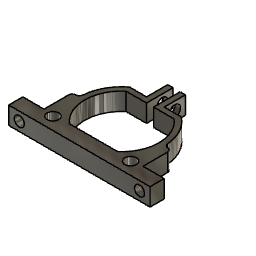
motor unite left v17 (Autodesk Fusion 360 archive; units mm, degrees)
design "motor mount back"
Autodesk Fusion 360 part; units mm, degrees
sketch "スケッチ1" plane through (0, 0, 0) normal (0, 0, 1) x (1, 0, 0)
  line L0 (-14, -12) -> (14, -12)
  line L1 (14, -12) -> (20, -12)
  line L2 (20, -12) -> (20, -8)
  line L3 (20, -8) -> (14, -8)
  line L4 (-14, -12) -> (-20, -12)
  line L5 (-20, -12) -> (-20, -8)
  line L6 (-20, -8) -> (-14, -8)
  line L7 (-14, -8) -> (-14, 0)
  line L8 (14, -8) -> (14, 0)
  circle A0 centre (11, -8.5) radius 1.65
  circle A1 centre (-11, -8.5) radius 1.65
  line L9 (0, 8) -> (-6.8007, 8)
  line L10 (0, 8) -> (6.8007, 8)
  line L11 (0, -8) -> (6.8007, -8)
  line L12 (0, -8) -> (-6.8007, -8)
  arc A2 (-6.8007, 8) -> (-6.8007, -8) centre (0, 0) ccw
  arc A3 (6.8007, -8) -> (6.8007, 8) centre (0, 0) ccw
  line L13 (-14, 0) -> (-12, 0)
  line L14 (12, 0) -> (14, 0)
  line L15 (0, 9.5) -> (7.3314, 9.5)
  line L16 (0, 9.5) -> (-7.3314, 9.5)
  arc A4 (-7.3314, 9.5) -> (-12, 0) centre (0, 0) ccw
  arc A5 (12, 0) -> (7.3314, 9.5) centre (0, 0) ccw
  line L17 (-1, 13.5) -> (-2.5, 13.5)
  line L18 (-2.5, 13.5) -> (-2.5, 9.5)
  line L19 (-1, 13.5) -> (-1, 8)
  line L20 (1, 13.5) -> (1, 8)
  line L21 (1, 13.5) -> (2.5, 13.5)
  line L22 (2.5, 13.5) -> (2.5, 9.5)
  dimension "d223" = 3.3
  constraint perpendicular L1 L2
  constraint perpendicular L4 L5
  constraint perpendicular L6 L7
  constraint perpendicular L3 L8
  constraint coincident A2.centre A3.centre
  constraint perpendicular L7 L13
  constraint perpendicular L8 L14
  constraint parallel L16 L17
  constraint coincident L16 L18.end
  constraint perpendicular L16 L18
  constraint coincident L9 L19.end
  constraint perpendicular L9 L19
  constraint coincident L10 L20.end
  constraint perpendicular L10 L20
  constraint perpendicular L20 L21
  constraint coincident L15 L22.end
  constraint perpendicular L15 L22
  measures "d223" diameter of A0
extrude "押し出し51" add sketch "スケッチ1" along normal blind 5 contours L0 L1 L2 L3 L4 L5 L6 L7 L8 L9 L10 L11 L12 A2 A3 L13 L14 L15 L16 A4 A5 L19 L20 | L16 L17 L18 L19 | L15 L20 L21 L22
extrude "押し出し52" add 2 faces at (-1.5, 13.5, 1.6667) (1.5, 13.5, 1.6667) along direction (0, 1, 0) blind 2
ref_plane "作業平面23" through (2.5, 12.5, 2.5) normal (1, 0, 0) x (0, 1, 0)
sketch "スケッチ26" plane through (2.5, 12.5, 2.5) normal (1, 0, 0) x (0, 1, 0)
  circle A0 centre (0, 0) radius 1.6
  constraint coincident A0.centre origin
extrude "押し出し53" cut sketch "スケッチ26" against normal blind 7
ref_plane "作業平面24" through (17, -8, 2.5) normal (0, 1, 0) x (-1, 0, 0)
sketch "スケッチ27" plane through (17, -8, 2.5) normal (0, 1, 0) x (1, 0, 0)
  circle A0 centre (0, 0) radius 1.6
  dimension "d265" = 3.2
  constraint coincident A0.centre origin
  measures "d265" diameter of A0
extrude "押し出し54" cut sketch "スケッチ27" against normal blind 5
ref_plane "作業平面25" through (-17, -8, 2.5) normal (0, 1, 0) x (-1, 0, 0)
sketch "スケッチ28" plane through (-17, -8, 2.5) normal (0, 1, 0) x (1, 0, 0)
  circle A0 centre (0, 0) radius 1.6
  dimension "d269" = 3.2
  constraint coincident A0.centre origin
  measures "d269" diameter of A0
extrude "押し出し55" cut sketch "スケッチ28" against normal blind 5
fillet "フィレット63" radius 1 1 edges at (-14, 0, 2.5)
fillet "フィレット64" radius 1 1 edges at (-12, 0, 2.5)
fillet "フィレット65" radius 1 1 edges at (12, 0, 2.5)
fillet "フィレット66" radius 1 1 edges at (14, 0, 2.5)
sketch "スケッチ29" plane through (0, -12, 0) normal (0, -1, 0) x (1, 0, 0)
  circle A0 centre (-17, 2.5) radius 1.6
  circle A1 centre (17, 2.5) radius 1.6
  line L0 (-20, 0) -> (20, 0)
  line L1 (20, 0) -> (20, 5)
  line L2 (20, 5) -> (-20, 5)
  line L3 (-20, 5) -> (-20, 0)
  circle A2 centre (-17, 2.5) radius 1.55
  circle A3 centre (17, 2.5) radius 1.55
  dimension "d280" = 3.1
  dimension "d281" = 3.1
  constraint concentric A0 A2
  constraint concentric A1 A3
  measures "d280" diameter of A2
  measures "d281" diameter of A3
extrude "押し出し56" add sketch "スケッチ29" against normal blind 4 contours A0 | A1
sketch "スケッチ30" plane through (0, -12, 0) normal (0, -1, 0) x (1, 0, 0)
  circle A0 centre (17, 2.5) radius 1.55
  circle A1 centre (-17, 2.5) radius 1.55
  line L0 (-20, 0) -> (20, 0)
  line L1 (20, 0) -> (20, 5)
  line L2 (20, 5) -> (-20, 5)
  line L3 (-20, 5) -> (-20, 0)
  circle A2 centre (-17, 2.5) radius 1.425
  circle A3 centre (17, 2.5) radius 1.425
  dimension "d284" = 2.85
  dimension "d285" = 2.85
  constraint concentric A1 A2
  constraint concentric A0 A3
  measures "d284" diameter of A2
  measures "d285" diameter of A3
extrude "押し出し57" add sketch "スケッチ30" against normal blind 4 contours A0 | A1

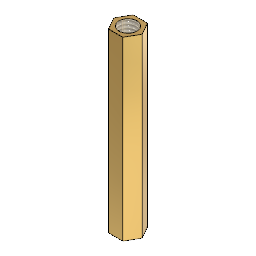
design "25mm m3 spacer"
Autodesk Fusion 360 part; units mm, degrees
sketch "スケッチ1" plane through (0, 0, 0) normal (0, 0, 1) x (1, 0, 0)
  circle A0 centre (0, 0) radius 1.5
  circle A1 centre (0, 0) radius 1.75
  line L0 (-1.0104, 1.75) -> (-2.0207, 0)
  line L1 (-2.0207, 0) -> (-1.0104, -1.75)
  line L2 (-1.0104, -1.75) -> (1.0104, -1.75)
  line L3 (1.0104, -1.75) -> (2.0207, 0)
  line L4 (2.0207, 0) -> (1.0104, 1.75)
  line L5 (1.0104, 1.75) -> (-1.0104, 1.75)
  constraint coincident A0.centre A1.centre
extrude "押し出し1" add sketch "スケッチ1" along normal blind 25
thread "ねじ1" "ISO Metric profile 3.0 M3x0.5 6H" major diameter 3.086 minor diameter 2.529 pitch 0.5 angle 60 resizes the face on face at (1.4925, -0.1494, 8.3333)
extrude "押し出し2" cut 1 faces at (1.3901, -0.7662, 25) along direction (0, 0, -1) blind 5
extrude "押し出し3" add 1 faces at (1.3901, -0.7662, 20) along direction (0, 0, 1) blind 10
extrude "押し出し4" cut 1 faces at (1.3901, -0.7662, 30) along direction (0, 0, -1) blind 5

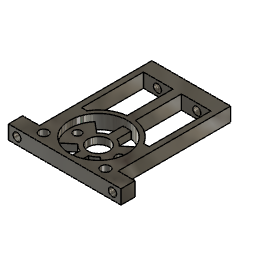
design "motor mount front"
Autodesk Fusion 360 part; units mm, degrees
sketch "スケッチ1" plane through (0, 0, 0) normal (0, 0, 1) x (1, 0, 0)
  circle A0 centre (0, 0) radius 10.25
  circle A1 centre (0, 0) radius 11.75
  circle A2 centre (0, 0) radius 3.75
  circle A3 centre (0, 0) radius 5.25
  line L0 (4.0217, 3.3746) -> (7.852, 6.5886)
  line L1 (4.0217, -3.3746) -> (7.852, -6.5886)
  line L2 (-1.5, 10.1396) -> (-1.5, 5.0312)
  line L3 (1.5, 10.1396) -> (1.5, 5.0312)
  line L4 (-1.5, -5.0312) -> (-1.5, -10.1396)
  line L5 (1.5, -10.1396) -> (1.5, -5.0312)
  line L6 (-4.0217, 3.3746) -> (-7.852, 6.5886)
  line L7 (-4.0217, -3.3746) -> (-7.852, -6.5886)
  circle A4 centre (-7.5, 0) radius 1.25
  circle A5 centre (7.5, 0) radius 1.25
  line L8 (-14, 20) -> (-14, -12)
  line L9 (-14, 20) -> (14, 20)
  line L10 (-14, -12) -> (14, -12)
  circle A6 centre (-11, -8.5) radius 1.5
  circle A7 centre (11, -8.5) radius 1.5
  line L11 (14, 20) -> (14, -12)
  line L12 (12, 6) -> (10.1026, 6)
  line L13 (-12, 6) -> (-10.1026, 6)
  line L14 (14, -12) -> (20, -12)
  line L15 (20, -12) -> (20, -8)
  line L16 (20, -8) -> (14, -8)
  line L17 (-14, -12) -> (-20, -12)
  line L18 (-20, -12) -> (-20, -8)
  line L19 (-20, -8) -> (-14, -8)
  line L20 (-12, 6) -> (-12, 15)
  line L21 (-12, 15) -> (12, 15)
  line L22 (12, 15) -> (12, 6)
  line L23 (-1.5, 15) -> (-1.5, 11.6539)
  line L24 (1.5, 15) -> (1.5, 11.6539)
  circle A8 centre (11, 17) radius 1.5
  circle A9 centre (-11, 17) radius 1.5
  constraint coincident A0.centre A1.centre
  constraint coincident A3 L0.start
  constraint coincident A0 L0.end
  constraint coincident A3 L1.start
  constraint coincident A0 L1.end
  constraint coincident A0 L2.start
  constraint coincident A3 L2.end
  constraint coincident A0 L3.start
  constraint coincident A3 L3.end
  constraint coincident A3 L4.start
  constraint coincident A0 L4.end
  constraint coincident A0 L5.start
  constraint coincident A3 L5.end
  constraint coincident A3 L6.start
  constraint coincident A0 L6.end
  constraint coincident A3 L7.start
  constraint coincident A0 L7.end
  constraint perpendicular L10 L11
  constraint coincident A1 L12.end
  constraint coincident A1 L13.end
  constraint perpendicular L11 L14
  constraint perpendicular L14 L15
  constraint coincident L11 L16.end
  constraint perpendicular L11 L16
  constraint perpendicular L8 L17
  constraint perpendicular L17 L18
  constraint coincident L8 L19.end
  constraint perpendicular L8 L19
  constraint perpendicular L13 L20
  constraint perpendicular L20 L21
  constraint perpendicular L12 L22
  constraint coincident A1 L23.end
  constraint perpendicular L12 L23
  constraint coincident L21 L24.start
  constraint coincident A1 L24.end
  constraint perpendicular L21 L24
extrude "押し出し29" add sketch "スケッチ1" along normal blind 5 contours A1 | A1 L21 L23 L24 | L8 L9 L10 L11 | L8 L17 L18 L19 | L11 L14 L15 L16 | A8 | A9
extrude "押し出し30" add sketch "スケッチ1" along normal blind 2.5 contours A0 A3 L0 L1 | A0 A3 L2 L3 | A3 | A0 A3 L4 L5 | A0 A3 L6 L7
thread "ねじ23" "ISO Metric profile 2.5 M2.5x0.45 6H" major diameter 2.58 minor diameter 2.0755 pitch 0.45 angle 60 resizes the face on face at (-6.2516, -0.0623, 1.6667)
thread "ねじ24" "ISO Metric profile 2.5 M2.5x0.45 6H" major diameter 2.58 minor diameter 2.0755 pitch 0.45 angle 60 resizes the face on face at (8.7484, -0.0623, 1.6667)
thread "ねじ25" "ISO Metric profile 3.0 M3x0.5 6H" major diameter 3.086 minor diameter 2.529 pitch 0.5 angle 60 resizes the face on face at (12.4981, -8.5748, 3.3333)
thread "ねじ26" "ISO Metric profile 3.0 M3x0.5 6H" major diameter 3.086 minor diameter 2.529 pitch 0.5 angle 60 resizes the face on face at (-9.5019, -8.5748, 3.3333)
ref_plane "作業平面14" through (-17, -8, 2.5) normal (0, 1, 0) x (-1, 0, 0)
sketch "スケッチ16" plane through (-17, -8, 2.5) normal (0, 1, 0) x (1, 0, 0)
  circle A0 centre (0, 0) radius 1.5
  dimension "d167" = 3
  constraint coincident A0.centre origin
  measures "d167" diameter of A0
extrude "押し出し32" cut sketch "スケッチ16" against normal blind 4
ref_plane "作業平面15" through (17, -8, 2.5) normal (0, 1, 0) x (-1, 0, 0)
sketch "スケッチ17" plane through (17, -8, 2.5) normal (0, 1, 0) x (1, 0, 0)
  circle A0 centre (0, 0) radius 1.5
  dimension "d171" = 3
  constraint coincident A0.centre origin
  measures "d171" diameter of A0
extrude "押し出し33" cut sketch "スケッチ17" against normal blind 4
thread "ねじ29" "ISO Metric profile 3.0 M3x0.5 6H" major diameter 3.086 minor diameter 2.529 pitch 0.5 angle 60 resizes the face on face at (-15.5075, -9.3333, 2.6494)
thread "ねじ30" "ISO Metric profile 3.0 M3x0.5 6H" major diameter 3.086 minor diameter 2.529 pitch 0.5 angle 60 resizes the face on face at (18.4925, -9.3333, 2.6494)
ref_plane "作業平面16" through (0, 20, 2.5) normal (0, 1, 0) x (-1, 0, 0)
sketch "スケッチ18" plane through (0, 20, 2.5) normal (0, 1, 0) x (1, 0, 0)
  line L0 (0, 0) -> (7, 0)
  line L1 (7, 0) -> (0, 0)
  line L2 (0, 0) -> (-7, 0)
  circle A0 centre (-7, 0) radius 1.5
  circle A1 centre (7, 0) radius 1.5
  dimension "d175" = 3
  dimension "d176" = 3
  constraint coincident L0.start L1.end
  constraint horizontal L0
  constraint parallel L0 L1
  constraint parallel L0 L2
  constraint coincident L2.end A0.centre
  constraint coincident L0.end L1.start
  measures "d175" diameter of A0
  measures "d176" diameter of A1
extrude "押し出し34" cut sketch "スケッチ18" against normal blind 5.5
thread "ねじ31" "ISO Metric profile 3.0 M3x0.5 6H" major diameter 3.086 minor diameter 2.529 pitch 0.5 angle 60 resizes the face on face at (8.4981, 16.6667, 2.5748)
thread "ねじ32" "ISO Metric profile 3.0 M3x0.5 6H" major diameter 3.086 minor diameter 2.529 pitch 0.5 angle 60 resizes the face on face at (-5.5075, 18.3333, 2.6494)
extrude "押し出し35" add 1 faces at (-12.0882, 20, 2.5) along direction (0, 1, 0) blind 3
extrude "押し出し36" cut 1 faces at (-2.9118, 15, 2.5) along direction (0, 1, 0) blind 3
extrude "押し出し37" cut 1 faces at (2.9118, 15, 2.5) along direction (0, 1, 0) blind 3
sketch "スケッチ19" plane through (0, -12, 0) normal (0, -1, 0) x (1, 0, 0)
  circle A0 centre (17, 2.5) radius 1.2645
  circle A1 centre (-17, 2.5) radius 1.2645
  line L0 (-20, 0) -> (20, 0)
  line L1 (20, 0) -> (20, 5)
  line L2 (20, 5) -> (-20, 5)
  line L3 (-20, 5) -> (-20, 0)
  circle A2 centre (17, 2.5) radius 1.75
  circle A3 centre (-17, 2.5) radius 1.75
  dimension "d195" = 3.5
  dimension "d196" = 3.5
  constraint concentric A0 A2
  constraint concentric A1 A3
  measures "d195" diameter of A2
  measures "d196" diameter of A3
extrude "押し出し38" cut sketch "スケッチ19" against normal blind 7 contours A2 | A3
sketch "スケッチ20" plane through (0, 0, 5) normal (0, 0, 1) x (-1, 0, 0)
  circle A0 centre (-11, 8.5) radius 1.2645
  line L0 (12, -6) -> (12, -18)
  line L1 (12, -18) -> (1.5, -18)
  line L2 (1.5, -18) -> (1.5, -11.6539)
  arc A1 (1.5, -11.6539) -> (10.1026, -6) centre (0, 0) ccw
  line L3 (10.1026, -6) -> (12, -6)
  line L4 (-1.5, -11.6539) -> (-1.5, -18)
  line L5 (-1.5, -18) -> (-12, -18)
  line L6 (-12, -18) -> (-12, -6)
  line L7 (-12, -6) -> (-10.1026, -6)
  arc A2 (-10.1026, -6) -> (-1.5, -11.6539) centre (0, 0) ccw
  circle A3 centre (11, 8.5) radius 1.2645
  circle A4 centre (0, 0) radius 10.25
  line L8 (20, 12) -> (-20, 12)
  line L9 (-20, 12) -> (-20, 8)
  line L10 (-20, 8) -> (-14, 8)
  line L11 (-14, 8) -> (-14, -23)
  line L12 (-14, -23) -> (14, -23)
  line L13 (14, -23) -> (14, 8)
  line L14 (14, 8) -> (20, 8)
  line L15 (20, 8) -> (20, 12)
  circle A5 centre (-11, 8.5) radius 1.75
  circle A6 centre (11, 8.5) radius 1.75
  dimension "d199" = 3.5
  dimension "d200" = 3.5
  constraint concentric A0 A5
  constraint concentric A3 A6
  measures "d199" diameter of A5
  measures "d200" diameter of A6
extrude "押し出し39" cut sketch "スケッチ20" against normal blind 12 contours A5 | A6
sketch "スケッチ21" plane through (0, 0, 2.5) normal (0, 0, 1) x (-1, 0, 0)
  circle A0 centre (-7.5, 0) radius 1.0377
  circle A1 centre (7.5, 0) radius 1.0377
  circle A2 centre (0, 0) radius 3.75
  line L0 (1.5, 5.0312) -> (1.5, 10.1396)
  arc A3 (1.5, 10.1396) -> (-1.5, 10.1396) centre (0, 0) ccw
  line L1 (-1.5, 10.1396) -> (-1.5, 5.0312)
  arc A4 (-1.5, 5.0312) -> (-4.0217, 3.3746) centre (0, 0) ccw
  line L2 (-4.0217, 3.3746) -> (-7.852, 6.5886)
  arc A5 (-7.852, 6.5886) -> (-7.852, -6.5886) centre (0, 0) ccw
  line L3 (-7.852, -6.5886) -> (-4.0217, -3.3746)
  arc A6 (-4.0217, -3.3746) -> (-1.5, -5.0312) centre (0, 0) ccw
  line L4 (-1.5, -5.0312) -> (-1.5, -10.1396)
  arc A7 (-1.5, -10.1396) -> (1.5, -10.1396) centre (0, 0) ccw
  line L5 (1.5, -10.1396) -> (1.5, -5.0312)
  arc A8 (1.5, -5.0312) -> (4.0217, -3.3746) centre (0, 0) ccw
  line L6 (4.0217, -3.3746) -> (7.852, -6.5886)
  arc A9 (7.852, -6.5886) -> (7.852, 6.5886) centre (0, 0) ccw
  line L7 (7.852, 6.5886) -> (4.0217, 3.3746)
  arc A10 (4.0217, 3.3746) -> (1.5, 5.0312) centre (0, 0) ccw
  circle A11 centre (7.5, 0) radius 1.35
  circle A12 centre (-7.5, 0) radius 1.35
  dimension "d203" = 2.7
  dimension "d204" = 2.7
  constraint concentric A1 A11
  constraint concentric A0 A12
  measures "d203" diameter of A11
  measures "d204" diameter of A12
extrude "押し出し40" cut sketch "スケッチ21" against normal blind 10 contours A11 | A12
sketch "スケッチ22" plane through (0, -12, 0) normal (0, -1, 0) x (1, 0, 0)
  circle A0 centre (-17, 2.5) radius 1.75
  circle A1 centre (17, 2.5) radius 1.75
  line L0 (-20, 0) -> (20, 0)
  line L1 (20, 0) -> (20, 5)
  line L2 (20, 5) -> (-20, 5)
  line L3 (-20, 5) -> (-20, 0)
  circle A2 centre (-17, 2.5) radius 1.75
  circle A3 centre (-17, 2.5) radius 1.65
  circle A4 centre (17, 2.5) radius 1.65
  dimension "d225" = 3.3
  dimension "d226" = 3.3
  constraint concentric A0 A2
  constraint concentric A0 A3
  constraint concentric A1 A4
  measures "d225" diameter of A3
  measures "d226" diameter of A4
extrude "押し出し45" add sketch "スケッチ22" against normal blind 4 contours A0 A2 | A1
sketch "スケッチ23" plane through (0, 0, 2.5) normal (0, 0, 1) x (-1, 0, 0)
  circle A0 centre (7.5, 0) radius 1.35
  circle A1 centre (-7.5, 0) radius 1.35
  circle A2 centre (0, 0) radius 3.75
  line L0 (1.5, 5.0312) -> (1.5, 10.1396)
  arc A3 (1.5, 10.1396) -> (-1.5, 10.1396) centre (0, 0) ccw
  line L1 (-1.5, 10.1396) -> (-1.5, 5.0312)
  arc A4 (-1.5, 5.0312) -> (-4.0217, 3.3746) centre (0, 0) ccw
  line L2 (-4.0217, 3.3746) -> (-7.852, 6.5886)
  arc A5 (-7.852, 6.5886) -> (-7.852, -6.5886) centre (0, 0) ccw
  line L3 (-7.852, -6.5886) -> (-4.0217, -3.3746)
  arc A6 (-4.0217, -3.3746) -> (-1.5, -5.0312) centre (0, 0) ccw
  line L4 (-1.5, -5.0312) -> (-1.5, -10.1396)
  arc A7 (-1.5, -10.1396) -> (1.5, -10.1396) centre (0, 0) ccw
  line L5 (1.5, -10.1396) -> (1.5, -5.0312)
  arc A8 (1.5, -5.0312) -> (4.0217, -3.3746) centre (0, 0) ccw
  line L6 (4.0217, -3.3746) -> (7.852, -6.5886)
  arc A9 (7.852, -6.5886) -> (7.852, 6.5886) centre (0, 0) ccw
  line L7 (7.852, 6.5886) -> (4.0217, 3.3746)
  arc A10 (4.0217, 3.3746) -> (1.5, 5.0312) centre (0, 0) ccw
  circle A11 centre (7.5, 0) radius 1.5
  circle A12 centre (-7.5, 0) radius 1.5
  dimension "d208" = 3
  dimension "d209" = 3
  constraint concentric A0 A11
  constraint concentric A1 A12
  measures "d208" diameter of A11
  measures "d209" diameter of A12
extrude "押し出し41" cut sketch "スケッチ23" against normal blind 6 contours A1 | A11 | A12
sketch "スケッチ24" plane through (0, 23, 0) normal (0, 1, 0) x (-1, 0, 0)
  circle A0 centre (-7, 2.5) radius 1.2645
  circle A1 centre (7, 2.5) radius 1.2645
  line L0 (-14, 0) -> (14, 0)
  line L1 (14, 0) -> (14, 5)
  line L2 (14, 5) -> (-14, 5)
  line L3 (-14, 5) -> (-14, 0)
  circle A2 centre (7, 2.5) radius 1.65
  circle A3 centre (-7, 2.5) radius 1.65
  dimension "d213" = 3.3
  dimension "d214" = 3.3
  constraint concentric A1 A2
  constraint concentric A0 A3
  measures "d213" diameter of A2
  measures "d214" diameter of A3
extrude "押し出し42" cut sketch "スケッチ24" against normal blind 8 contours A2 | A3
sketch "スケッチ25" plane through (0, 0, 5) normal (0, 0, 1) x (-1, 0, 0)
  circle A0 centre (11, 8.5) radius 1.75
  circle A1 centre (-11, 8.5) radius 1.75
  line L0 (12, -6) -> (12, -18)
  line L1 (12, -18) -> (1.5, -18)
  line L2 (1.5, -18) -> (1.5, -11.6539)
  arc A2 (1.5, -11.6539) -> (10.1026, -6) centre (0, 0) ccw
  line L3 (10.1026, -6) -> (12, -6)
  line L4 (-1.5, -11.6539) -> (-1.5, -18)
  line L5 (-1.5, -18) -> (-12, -18)
  line L6 (-12, -18) -> (-12, -6)
  line L7 (-12, -6) -> (-10.1026, -6)
  arc A3 (-10.1026, -6) -> (-1.5, -11.6539) centre (0, 0) ccw
  circle A4 centre (0, 0) radius 10.25
  line L8 (20, 12) -> (-20, 12)
  line L9 (-20, 12) -> (-20, 8)
  line L10 (-20, 8) -> (-14, 8)
  line L11 (-14, 8) -> (-14, -23)
  line L12 (-14, -23) -> (14, -23)
  line L13 (14, -23) -> (14, 8)
  line L14 (14, 8) -> (20, 8)
  line L15 (20, 8) -> (20, 12)
  circle A5 centre (11, 8.5) radius 1.65
  circle A6 centre (-11, 8.5) radius 1.65
  dimension "d217" = 3.3
  dimension "d218" = 3.3
  constraint concentric A0 A5
  constraint concentric A1 A6
  measures "d217" diameter of A5
  measures "d218" diameter of A6
extrude "押し出し43" add sketch "スケッチ25" against normal blind 5 contours A0 | A1
sketch "スケッチ26" plane through (0, 0, 2.5) normal (0, 0, 1) x (-1, 0, 0)
  circle A0 centre (-7.5, 0) radius 1.5
  circle A1 centre (7.5, 0) radius 1.5
  circle A2 centre (0, 0) radius 3.75
  line L0 (1.5, 5.0312) -> (1.5, 10.1396)
  arc A3 (1.5, 10.1396) -> (-1.5, 10.1396) centre (0, 0) ccw
  line L1 (-1.5, 10.1396) -> (-1.5, 5.0312)
  arc A4 (-1.5, 5.0312) -> (-4.0217, 3.3746) centre (0, 0) ccw
  line L2 (-4.0217, 3.3746) -> (-7.852, 6.5886)
  arc A5 (-7.852, 6.5886) -> (-7.852, -6.5886) centre (0, 0) ccw
  line L3 (-7.852, -6.5886) -> (-4.0217, -3.3746)
  arc A6 (-4.0217, -3.3746) -> (-1.5, -5.0312) centre (0, 0) ccw
  line L4 (-1.5, -5.0312) -> (-1.5, -10.1396)
  arc A7 (-1.5, -10.1396) -> (1.5, -10.1396) centre (0, 0) ccw
  line L5 (1.5, -10.1396) -> (1.5, -5.0312)
  arc A8 (1.5, -5.0312) -> (4.0217, -3.3746) centre (0, 0) ccw
  line L6 (4.0217, -3.3746) -> (7.852, -6.5886)
  arc A9 (7.852, -6.5886) -> (7.852, 6.5886) centre (0, 0) ccw
  line L7 (7.852, 6.5886) -> (4.0217, 3.3746)
  arc A10 (4.0217, 3.3746) -> (1.5, 5.0312) centre (0, 0) ccw
  circle A11 centre (-7.5, 0) radius 1.4
  circle A12 centre (7.5, 0) radius 1.4
  dimension "d221" = 2.8
  dimension "d222" = 2.8
  constraint concentric A0 A11
  constraint concentric A1 A12
  measures "d221" diameter of A11
  measures "d222" diameter of A12
extrude "押し出し44" add sketch "スケッチ26" against normal blind 2.5 contours A0 | A1
sketch "スケッチ27" plane through (0, -12, 0) normal (0, -1, 0) x (1, 0, 0)
  circle A0 centre (-17, 2.5) radius 1.65
  circle A1 centre (17, 2.5) radius 1.65
  line L0 (-20, 0) -> (20, 0)
  line L1 (20, 0) -> (20, 5)
  line L2 (20, 5) -> (-20, 5)
  line L3 (-20, 5) -> (-20, 0)
  circle A2 centre (17, 2.5) radius 1.6
  circle A3 centre (-17, 2.5) radius 1.6
  dimension "d230" = 3.2
  dimension "d231" = 3.2
  constraint concentric A1 A2
  constraint concentric A0 A3
  measures "d230" diameter of A2
  measures "d231" diameter of A3
extrude "押し出し46" add sketch "スケッチ27" against normal blind 4 contours A0 | A1
sketch "スケッチ28" plane through (0, 23, 0) normal (0, 1, 0) x (-1, 0, 0)
  circle A0 centre (-7, 2.5) radius 1.65
  circle A1 centre (7, 2.5) radius 1.65
  line L0 (-14, 0) -> (14, 0)
  line L1 (14, 0) -> (14, 5)
  line L2 (14, 5) -> (-14, 5)
  line L3 (-14, 5) -> (-14, 0)
  circle A2 centre (-7, 2.5) radius 1.6
  dimension "d234" = 3.2
  constraint concentric A0 A2
  measures "d234" diameter of A2
extrude "押し出し47" add sketch "スケッチ28" against normal blind 5 contours A0
sketch "スケッチ29" plane through (0, 23, 0) normal (0, 1, 0) x (-1, 0, 0)
  circle A0 centre (-7, 2.5) radius 1.6
  circle A1 centre (7, 2.5) radius 1.65
  line L0 (-14, 0) -> (14, 0)
  line L1 (14, 0) -> (14, 5)
  line L2 (14, 5) -> (-14, 5)
  line L3 (-14, 5) -> (-14, 0)
  circle A2 centre (7, 2.5) radius 1.6
  dimension "d237" = 3.2
  constraint concentric A1 A2
  measures "d237" diameter of A2
extrude "押し出し48" add sketch "スケッチ29" against normal blind 5 contours A1
extrude "押し出し49" add 1 faces at (12.2, 23, 2.5) along direction (0, 1, 0) blind 10
extrude "押し出し50" cut 2 faces at (-2.8, 18, 2.5) (2.8, 18, 2.5) along direction (0, 1, 0) blind 10
sketch "スケッチ31" plane through (0, -12, 0) normal (0, -1, 0) x (1, 0, 0)
  circle A0 centre (-17, 2.5) radius 1.6
  circle A1 centre (17, 2.5) radius 1.6
  line L0 (-20, 0) -> (20, 0)
  line L1 (20, 0) -> (20, 5)
  line L2 (20, 5) -> (-20, 5)
  line L3 (-20, 5) -> (-20, 0)
  circle A2 centre (-17, 2.5) radius 1.55
  dimension "d247" = 3.1
  constraint concentric A0 A2
  measures "d247" diameter of A2
extrude "押し出し51" add sketch "スケッチ31" against normal blind 5 contours A0
sketch "スケッチ32" plane through (0, -12, 0) normal (0, -1, 0) x (1, 0, 0)
  circle A0 centre (-17, 2.5) radius 1.55
  circle A1 centre (17, 2.5) radius 1.6
  line L0 (-20, 0) -> (20, 0)
  line L1 (20, 0) -> (20, 5)
  line L2 (20, 5) -> (-20, 5)
  line L3 (-20, 5) -> (-20, 0)
  circle A2 centre (17, 2.5) radius 1.55
  dimension "d250" = 3.1
  constraint concentric A1 A2
  measures "d250" diameter of A2
extrude "押し出し52" add sketch "スケッチ32" against normal blind 5 contours A1
extrude "押し出し53" cut 1 faces at (-18.3867, -7, 3.256) along direction (0, -1, 0) blind 1
extrude "押し出し54" cut 1 faces at (18.3867, -7, 3.256) along direction (0, -1, 0) blind 1
sketch "スケッチ33" plane through (0, 33, 0) normal (0, 1, 0) x (-1, 0, 0)
  circle A0 centre (7, 2.5) radius 1.6
  circle A1 centre (-7, 2.5) radius 1.6
  line L0 (-14, 0) -> (14, 0)
  line L1 (14, 0) -> (14, 5)
  line L2 (14, 5) -> (-14, 5)
  line L3 (-14, 5) -> (-14, 0)
  circle A2 centre (-7, 2.5) radius 1.55
  circle A3 centre (7, 2.5) radius 1.55
  dimension "d257" = 3.1
  dimension "d258" = 3.1
  constraint concentric A1 A2
  constraint concentric A0 A3
  measures "d257" diameter of A2
  measures "d258" diameter of A3
extrude "押し出し55" add sketch "スケッチ33" against normal blind 5 contours A0 | A1
extrude "押し出し56" add 1 faces at (-19.5167, -8, 2.5) along direction (0, 1, 0) blind 1
extrude "押し出し57" add 1 faces at (19.5167, -8, 2.5) along direction (0, 1, 0) blind 1
sketch "スケッチ34" plane through (0, -12, 0) normal (0, -1, 0) x (1, 0, 0)
  circle A0 centre (17, 2.5) radius 1.55
  circle A1 centre (-17, 2.5) radius 1.55
  line L0 (-20, 0) -> (20, 0)
  line L1 (20, 0) -> (20, 5)
  line L2 (20, 5) -> (-20, 5)
  line L3 (-20, 5) -> (-20, 0)
  circle A2 centre (-17, 2.5) radius 1.425
  circle A3 centre (17, 2.5) radius 1.425
  dimension "d265" = 2.85
  dimension "d266" = 2.85
  constraint concentric A1 A2
  constraint concentric A0 A3
  measures "d265" diameter of A2
  measures "d266" diameter of A3
extrude "押し出し58" add sketch "スケッチ34" against normal blind 5 contours A0 | A1
sketch "スケッチ35" plane through (0, 33, 0) normal (0, 1, 0) x (-1, 0, 0)
  circle A0 centre (7, 2.5) radius 1.55
  circle A1 centre (-7, 2.5) radius 1.55
  line L0 (-14, 0) -> (14, 0)
  line L1 (14, 0) -> (14, 5)
  line L2 (14, 5) -> (-14, 5)
  line L3 (-14, 5) -> (-14, 0)
  circle A2 centre (7, 2.5) radius 1.425
  circle A3 centre (-7, 2.5) radius 1.425
  dimension "d269" = 2.85
  dimension "d270" = 2.85
  constraint concentric A0 A2
  constraint concentric A1 A3
  measures "d269" diameter of A2
  measures "d270" diameter of A3
extrude "押し出し59" add sketch "スケッチ35" against normal blind 5 contours A0 | A1

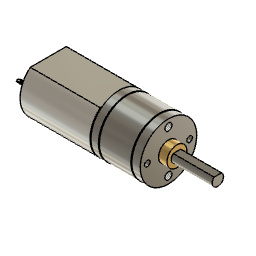
design "pololu 78:1 motor"
Autodesk Fusion 360 part; units mm, degrees
sketch "スケッチ1" plane through (0, 0, 0) normal (0, 0, 1) x (1, 0, 0)
  circle A0 centre (0, 0) radius 10
  line L0 (0, 0) -> (0, 7.7)
  line L1 (0, 7.7) -> (-6.3804, 7.7)
  line L2 (0, 7.7) -> (6.3804, 7.7)
  line L3 (0, 0) -> (0, -7.7)
  line L4 (0, -7.7) -> (6.3804, -7.7)
  line L5 (-6.3804, -7.7) -> (0, -7.7)
  dimension "d1" = 20
  dimension "d2" = 7.7
  dimension "d3" = 7.7
  constraint coincident A0.centre L0.start
  constraint vertical L0
  constraint coincident A0 L1.end
  constraint perpendicular L0 L1
  constraint coincident A0 L2.end
  constraint perpendicular L0 L2
  constraint perpendicular L2 L3
  constraint coincident A0 L4.end
  constraint perpendicular L3 L4
  constraint coincident A0 L5.start
  constraint perpendicular L3 L5
  measures "d1" diameter of A0
  measures "d2" distance of A0.centre L0.end
  measures "d3" distance of A0.centre L3.end
extrude "押し出し1" add sketch "スケッチ1" along normal blind 25.1 contours A0 L0 L2 L3 L4 | A0 L0 L1 L3 L5 makes body 1
ref_plane "作業平面1" through (0, 0, 25.1) normal (0, 0, 1) x (1, 0, 0)
sketch "スケッチ2" plane through (0, 0, 25.1) normal (0, 0, 1) x (1, 0, 0)
  circle A0 centre (0, 0) radius 10
  constraint coincident A0.centre origin
chamfer "面取り1" distance 0.3 angle 45 1 edges at (-10, 0, 25.1) on bodies 1
chamfer "面取り2" distance 0.3 angle 45 1 edges at (0.2406, -7.7, 25.1) on bodies 1
chamfer "面取り3" distance 0.3 angle 45 1 edges at (9.9974, 0.2288, 25.1) on bodies 1
chamfer "面取り4" distance 0.3 angle 45 1 edges at (0, 7.7, 25.1) on bodies 1
ref_plane "作業平面2" through (0, 0, 25.1) normal (0, 0, 1) x (1, 0, 0)
sketch "スケッチ3" plane through (0, 0, 25.1) normal (0, 0, 1) x (1, 0, 0)
  circle A0 centre (0, 0) radius 10
  constraint coincident A0.centre origin
ref_plane "作業平面3" through (0, 0, 25.1) normal (0, 0, 1) x (1, 0, 0)
sketch "スケッチ4" plane through (0, 0, 25.1) normal (0, 0, 1) x (1, 0, 0)
  circle A0 centre (0, 0) radius 10
  constraint coincident A0.centre origin
ref_plane "作業平面5" through (0, 0, 25.1) normal (0, 0, 1) x (1, 0, 0)
sketch "スケッチ5" plane through (0, 0, 25.1) normal (0, 0, 1) x (1, 0, 0)
  circle A0 centre (0, 0) radius 10
  constraint coincident A0.centre origin
extrude "押し出し5" add sketch "スケッチ5" along normal blind 3 bodies 1
chamfer "面取り6" distance 0.3 angle 45 1 edges at (-9.3233, -3.6162, 28.1) on bodies 1
ref_plane "作業平面6" through (0, 0, 28.1) normal (0, 0, 1) x (1, 0, 0)
sketch "スケッチ6" plane through (0, 0, 28.1) normal (0, 0, 1) x (1, 0, 0)
  circle A0 centre (0, 0) radius 10
  constraint coincident A0.centre origin
extrude "押し出し6" add sketch "スケッチ6" along normal blind 11.5 bodies 1
chamfer "面取り7" distance 0.3 angle 45 1 edges at (-9.3233, -3.6162, 39.6) on bodies 1
ref_plane "作業平面8" through (0, 0, 39.6) normal (0, 0, 1) x (1, 0, 0)
sketch "スケッチ7" plane through (0, 0, 39.6) normal (0, 0, 1) x (1, 0, 0)
  circle A0 centre (0, 0) radius 10
  constraint coincident A0.centre origin
extrude "押し出し7" add sketch "スケッチ7" along normal blind 3 bodies 1
ref_plane "作業平面9" through (0, 0, 42.6) normal (0, 0, 1) x (1, 0, 0)
sketch "スケッチ8" plane through (0, 0, 42.6) normal (0, 0, 1) x (1, 0, 0)
  circle A0 centre (0, 0) radius 3.5
  dimension "d34" = 7
  constraint coincident A0.centre origin
  measures "d34" diameter of A0
extrude "押し出し8" add sketch "スケッチ8" along normal blind 3 bodies 1
ref_plane "作業平面10" through (0, 0, 45.6) normal (0, 0, 1) x (1, 0, 0)
sketch "スケッチ9" plane through (0, 0, 45.6) normal (0, 0, 1) x (1, 0, 0)
  circle A0 centre (0, 0) radius 2
  line L0 (0, -2) -> (0, 1.5)
  line L1 (0, 1.5) -> (1.3229, 1.5)
  line L2 (-1.3229, 1.5) -> (0, 1.5)
  dimension "d38" = 4
  dimension "d39" = 3.5
  constraint coincident A0.centre origin
  constraint coincident A0 L0.start
  constraint vertical L0
  constraint coincident A0 L1.end
  constraint perpendicular L0 L1
  constraint coincident A0 L2.start
  constraint perpendicular L0 L2
  measures "d38" diameter of A0
  measures "d39" distance of L0.start L0.end
sketch "スケッチ10" plane through (0, 0, 46.6) normal (0, 0, 1) x (-1, 0, 0)
ref_plane "作業平面11" through (0, 0, 45.6) normal (0, 0, 1) x (1, 0, 0)
sketch "スケッチ11" plane through (0, 0, 45.6) normal (0, 0, 1) x (1, 0, 0)
  circle A0 centre (0, 0) radius 2
  line L0 (0, -2) -> (0, 1.5)
  line L1 (0, 1.5) -> (-1.3229, 1.5)
  line L2 (0, 1.5) -> (1.3229, 1.5)
  dimension "d43" = 3.5
  constraint coincident A0.centre origin
  constraint coincident A0 L0.start
  constraint vertical L0
  constraint coincident A0 L1.end
  constraint perpendicular L0 L1
  constraint coincident A0 L2.end
  constraint perpendicular L0 L2
  measures "d43" distance of L0.start L0.end
extrude "押し出し10" add sketch "スケッチ11" along normal blind 14.5 contours A0 L0 L2 | A0 L0 L1 bodies 1
ref_plane "作業平面12" through (0, 0, 0) normal (0, 0, 1) x (1, 0, 0)
sketch "スケッチ12" plane through (0, 0, 0) normal (0, 0, 1) x (1, 0, 0)
  circle A0 centre (0, 0) radius 3.1
  dimension "d47" = 6.2
  constraint coincident A0.centre origin
  measures "d47" diameter of A0
extrude "押し出し11" add sketch "スケッチ12" against normal blind 2.1 bodies 1
ref_plane "作業平面13" through (0, 0, -2.1) normal (0, 0, -1) x (-1, 0, 0)
sketch "スケッチ13" plane through (0, 0, -2.1) normal (0, 0, -1) x (1, 0, 0)
  circle A0 centre (0, 0) radius 1
  dimension "d51" = 2
  constraint coincident A0.centre origin
  measures "d51" diameter of A0
extrude "押し出し12" add sketch "スケッチ13" along normal blind 6 bodies 1
ref_plane "作業平面14" through (0, 0, 0) normal (0, 0, -1) x (-1, 0, 0)
sketch "スケッチ14" plane through (0, 0, 0) normal (0, 0, -1) x (1, 0, 0)
sketch "スケッチ15" plane through (0, 0, 0) normal (0, 0, -1) x (1, 0, 0)
  circle A0 centre (0, 0) radius 3.1
  line L0 (-6.3804, -7.7) -> (6.3804, -7.7)
  arc A1 (6.3804, -7.7) -> (6.3804, 7.7) centre (0, 0) ccw
  line L1 (6.3804, 7.7) -> (-6.3804, 7.7)
  arc A2 (-6.3804, 7.7) -> (-6.3804, -7.7) centre (0, 0) ccw
ref_plane "作業平面15" through (0, 0, 0) normal (0, 0, -1) x (1, 0, 0)
sketch "スケッチ16" plane through (0, 0, 0) normal (0, 0, -1) x (1, 0, 0)
  arc A0 (10, 0) -> (9.3969, 3.4202) centre (0, 0) ccw
  line L0 (0, 0) -> (10, 0) construction
  line L1 (0, 0) -> (9.3969, 3.4202) construction
  line L2 (0, 0) -> (6.2959, 2.2915)
  line L3 (6.2959, 2.2915) -> (-6.2959, -2.2915)
  line L4 (6.2959, 2.2915) -> (8.1753, 2.9756)
  line L5 (8.1753, 2.9756) -> (8.2779, 2.6937)
  line L6 (8.2779, 2.6937) -> (6.3985, 2.0096)
  line L7 (6.3985, 2.0096) -> (6.2959, 2.2915)
  line L8 (-6.2959, -2.2915) -> (-8.1753, -2.9756)
  line L9 (-8.1753, -2.9756) -> (-8.2779, -2.6937)
  line L10 (-8.2779, -2.6937) -> (-6.3985, -2.0096)
  line L11 (-6.3985, -2.0096) -> (-6.2959, -2.2915)
  dimension "d57" = 20
  dimension "d58" = 6.7
  dimension "d59" = 13.4
  dimension "d60" = 2
  dimension "d61" = 0.3
  dimension "d62" = 0.3
  constraint coincident A0.centre L0.start
  constraint parallel L1 L2
  constraint parallel L1 L3
  constraint perpendicular L4 L5
  constraint parallel L4 L6
  constraint parallel L5 L7
  constraint coincident L1 L4.end
  constraint perpendicular L8 L9
  constraint parallel L8 L10
  constraint parallel L9 L11
  constraint parallel L3 L8
  measures "d57" angle of L0 L1
  measures "d58" distance of A0.centre L2.end
  measures "d59" distance of L2.end L3.end
  measures "d60" distance of L2.end L4.end
  measures "d61" distance of L2.end L6.end
  measures "d62" distance of L3.end L10.end
extrude "押し出し13" add sketch "スケッチ16" along normal blind 3.6 bodies 1
ref_plane "作業平面16" through (-7.3382, 2.3516, -1.8) normal (-0.34202, -0.939693, 0) x (-0.939693, 0.34202, 0)
sketch "スケッチ17" plane through (-7.3382, 2.3516, -1.8) normal (-0.34202, -0.939693, 0) x (-0.939693, 0.34202, 0)
  line L0 (-14.4, -1.8) -> (-16.4, 1.8)
  line L1 (-14.4, 1.8) -> (-16.4, -1.8)
  circle A0 centre (-15.4, 0) radius 0.75
  dimension "d66" = 1.5
  constraint midpoint L0 A0.centre
  measures "d66" diameter of A0
extrude "押し出し14" cut sketch "スケッチ17" against normal blind 4 bodies 1
ref_plane "作業平面17" through (-7.3382, 2.3516, -1.8) normal (-0.34202, -0.939693, 0) x (-0.939693, 0.34202, 0)
sketch "スケッチ18" plane through (-7.3382, 2.3516, -1.8) normal (-0.34202, -0.939693, 0) x (-0.939693, 0.34202, 0)
  line L0 (-1, -1.8) -> (1, 1.8)
  line L1 (-1, 1.8) -> (1, -1.8)
  circle A0 centre (0, 0) radius 0.75
  dimension "d70" = 1.5
  constraint coincident A0.centre origin
  measures "d70" diameter of A0
extrude "押し出し15" cut sketch "スケッチ18" against normal blind 4 bodies 1
fillet "フィレット1" radius 1 1 edges at (8.2266, -2.8346, -3.6) on bodies 1
fillet "フィレット2" radius 1 1 edges at (6.3472, -2.1506, -3.6) on bodies 1
fillet "フィレット3" radius 1 1 edges at (-8.2266, 2.8346, -3.6) on bodies 1
fillet "フィレット4" radius 1 1 edges at (-6.3472, 2.1506, -3.6) on bodies 1
ref_plane "作業平面18" through (0, 0, 42.6) normal (0, 0, 1) x (1, 0, 0)
sketch "スケッチ19" plane through (0, 0, 42.6) normal (0, 0, 1) x (1, 0, 0)
  line L0 (0, 0) -> (7.5, 0)
  circle A0 centre (7.5, 0) radius 1
  line L1 (0, 0) -> (-7.5, 0)
  circle A1 centre (-7.5, 0) radius 1
  dimension "d78" = 7.5
  dimension "d79" = 2
  dimension "d80" = 7.5
  dimension "d81" = 2
  constraint coincident L0.start L1.start
  constraint horizontal L0
  constraint coincident L0.end A0.centre
  constraint parallel L0 L1
  constraint coincident L1.end A1.centre
  measures "d78" distance of L0.start L0.end
  measures "d79" diameter of A0
  measures "d80" distance of L0.start L1.end
  measures "d81" diameter of A1
extrude "押し出し16" cut sketch "スケッチ19" against normal blind 3 bodies 1
ref_plane "作業平面19" through (0, 0, 42.6) normal (0, 0, 1) x (1, 0, 0)
sketch "スケッチ20" plane through (0, 0, 42.6) normal (0, 0, 1) x (1, 0, 0)
  line L0 (0, 0) -> (0, 7.5)
  circle A0 centre (0, 7.5) radius 1.5
  line L1 (0, 0) -> (0, -7.5)
  circle A1 centre (0, -7.5) radius 1.5
  dimension "d85" = 7.5
  dimension "d86" = 3
  dimension "d87" = 7.5
  dimension "d88" = 3
  constraint coincident L0.start L1.start
  constraint vertical L0
  constraint coincident L0.end A0.centre
  constraint parallel L0 L1
  constraint coincident L1.end A1.centre
  measures "d85" distance of L0.start L0.end
  measures "d86" diameter of A0
  measures "d87" distance of L0.start L1.end
  measures "d88" diameter of A1
extrude "押し出し17" cut sketch "スケッチ20" against normal blind 6 bodies 1
thread "ねじ1" "ISO Metric profile 3.0 M3x0.5 6H" major diameter 3.086 minor diameter 2.529 pitch 0.5 angle 60 resizes the face on face at (1.4925, 7.6494, 40.6) on bodies 1
thread "ねじ2" "ISO Metric profile 3.0 M3x0.5 6H" major diameter 3.086 minor diameter 2.529 pitch 0.5 angle 60 resizes the face on face at (1.4925, -7.3506, 40.6) on bodies 1
move_body "移動1" bodies 1 to x (0, 0, -1) y (0, 1, 0) z (1, 0, 0) at (-17.2978, 0, 10.0267)
move_body "移動2" bodies 1 to x (1, 0, 0) y (0, 1, 0) z (0, 0, 1) at (0, 0, 5)
move_body "移動3" bodies 1 to x (1, 0, 0) y (0, 0, 1) z (0, -1, 0) at (0, -4.9733, 15.0267)
move_body "移動4" bodies 1 to x (1, 0, 0) y (0, 1, 0) z (0, 0, 1) at (0, 0, 5)
extrude "押し出し18" cut 1 faces at (-25.3978, -19.7064, 19.8074) along direction (1, 0, 0) blind 7 on bodies 1 bodies 1
extrude "押し出し19" cut 1 faces at (-19.3978, -17.6153, 19.823) along direction (1, 0, 0) blind 2 on bodies 1 bodies 1
extrude "押し出し20" cut 1 faces at (-18.3978, -19.7064, 19.8074) along direction (1, 0, 0) blind 1 on bodies 1 bodies 1
extrude "押し出し21" cut 1 faces at (-17.3978, -20.5167, 20.0285) along direction (1, 0, 0) up to surface (0.1 mm away) on bodies 1 bodies 1
ref_plane "作業平面20" through (7.8022, -20, 20.0267) normal (-1, 0, 0) x (0, -1, 0)
split "分割1" by plane through (7.8022, -20, 20.0267) normal (-1, 0, 0) bodies 1 makes body 2 at (-9.0311, -12.2466, 13.7112)
ref_plane "作業平面21" through (25.3022, -20, 20.0267) normal (1, 0, 0) x (0, 1, 0)
split "分割2" by plane through (25.3022, -20, 20.0267) normal (1, 0, 0) bodies 1 makes body 3 at (37.9689, -21.9487, 19.5766)
ref_plane "作業平面22" through (28.3022, -20, 20.0267) normal (1, 0, 0) x (0, 1, 0)
split "分割3" by plane through (28.3022, -20, 20.0267) normal (1, 0, 0) bodies 3 makes body 4 at (37.9689, -21.9487, 19.5766)
extrude "押し出し4" [suppressed]
chamfer "面取り5" [suppressed]
ref_plane "作業平面4" through (0, 0, 29.1) normal (0, 0, 1) x (1, 0, 0)
extrude "押し出し3" [suppressed]
extrude "押し出し2" [suppressed]

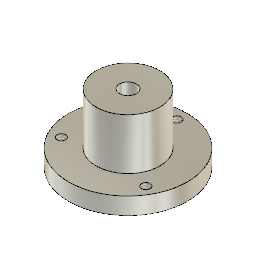
design "wheel hub"
Autodesk Fusion 360 part; units mm, degrees
sketch "スケッチ1" plane through (0, 0, 0) normal (0, 0, 1) x (1, 0, 0)
  circle A0 centre (0, 0) radius 14
  circle A1 centre (0, 0) radius 7.5
  circle A2 centre (0, 0) radius 2
  circle A3 centre (0, 0) radius 11.5
  arc A4 (9.959292, -5.75) -> (0, 11.5) centre (0, 0) ccw
  line L0 (0, 0) -> (9.959292, -5.75) construction
  line L1 (0, 0) -> (0, 11.5) construction
  arc A5 (0, 11.5) -> (-9.959292, -5.75) centre (0, 0) ccw
  line L2 (0, 0) -> (0, 11.5) construction
  line L3 (0, 0) -> (-9.959292, -5.75) construction
  circle A6 centre (0, 11.5) radius 1.25
  circle A7 centre (9.959292, -5.75) radius 1.25
  circle A8 centre (-9.959292, -5.75) radius 1.25
  dimension "d5" = 120
  dimension "d6" = 120
  dimension "d7" = 2.5
  dimension "d8" = 2.5
  dimension "d9" = 2.5
  constraint coincident A0.centre A1.centre
  constraint coincident A3 A4.end
  constraint coincident A4.end L1.end
  measures "d5" angle of L0 L1
  measures "d6" angle of L2 L3
  measures "d7" diameter of A6
  measures "d8" diameter of A7
  measures "d9" diameter of A8
extrude "押し出し1" add sketch "スケッチ1" along normal blind 4 contours A0 | A3 A4 A5 A6 A7 A8 picked at (3.710126, 12.603162) picked at (1.820316, 9.688085)
extrude "押し出し2" add sketch "スケッチ1" along normal blind 16 contours A1 picked at (5.631298, -0.471967)
ref_plane "作業平面1" through (-6.495191, 3.75, 11.585392) normal (-0.866025, 0.5, 0) x (0.5, 0.866025, 0)
sketch "スケッチ2" plane through (-6.495191, 3.75, 11.585392) normal (-0.866025, 0.5, 0) x (0.5, 0.866025, 0)
  line L0 (0, 11.585001) -> (0, 3.585001)
  circle A0 centre (0, 3.585001) radius 2
  dimension "d15" = 8
  dimension "d16" = 4
  constraint vertical L0
  measures "d16" diameter of A0
extrude "押し出し3" cut sketch "スケッチ2" against normal blind 7.5 contours A0 picked at (0.342132, 3.616673)
thread "ねじ1" "ISO Metric profile 4.0 M4x0.7 6H" major diameter 4.1095 minor diameter 3.332 pitch 0.7 angle 60 resizes the face on face at (-3.19291, -0.457664, 7.830887)
thread "ねじ2" "ISO Metric profile 2.5 M2.5x0.45 6H" major diameter 2.58 minor diameter 2.0755 pitch 0.45 angle 60 resizes the face on face at (-8.710846, -5.687693, 1.333333)
thread "ねじ3" "ISO Metric profile 2.5 M2.5x0.45 6H" major diameter 2.58 minor diameter 2.0755 pitch 0.45 angle 60 resizes the face on face at (1.248446, 11.562307, 1.333333)
thread "ねじ4" "ISO Metric profile 2.5 M2.5x0.45 6H" major diameter 2.58 minor diameter 2.0755 pitch 0.45 angle 60 resizes the face on face at (11.207738, -5.687693, 1.333333)
